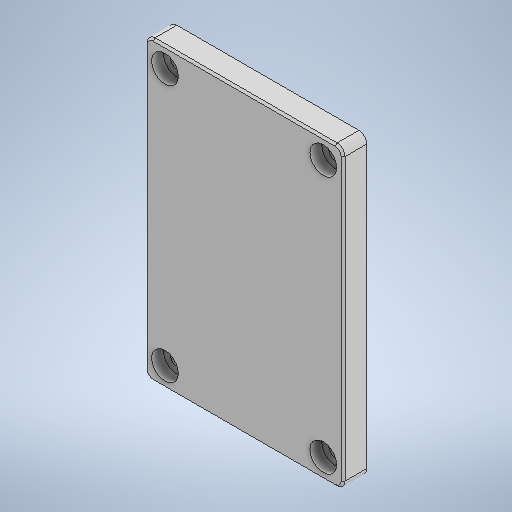
# Autodesk Inventor part: PCB_Cover
Saved by Autodesk Inventor 2025.3 (Build 293356000, 356)
## iProperties
Created: 2025-11-23
Part Number: PCB_Cover
Material: Generic
Document SubType Name: Modeling
Designer: Wula
Density: 1 g/cm^3
Appearance: Default
Author: Wula
Autodesk Inventor part; units mm, degrees
ref_plane "YZ Plane" through (0, 0, 0) normal (1, 0, 0) x (0, 1, 0)
ref_plane "XZ Plane" through (0, 0, 0) normal (0, 1, 0) x (-1, 0, 0)
ref_plane "XY Plane" through (0, 0, 0) normal (0, 0, 1) x (1, 0, 0)
sketch "Sketch1" plane through (0, 0, 0) normal (0, 1, 0) x (-1, 0, 0)
  line L0 (-50, 75) -> (50, 75)
  line L1 (50, 75) -> (50, -75)
  line L2 (50, -75) -> (-50, -75)
  line L3 (-50, -75) -> (-50, 75)
  line L4 (-50, 75) -> (50, -75) construction
  line L5 (50, 75) -> (-50, -75) construction
  point P0 (0, 0)
  dimension "d0" = 150
  dimension "d1" = 100
  constraints: 12 end point, 2 midpoint, 2 parallel, 1 horizontal, 1 perpendicular
  measures "d0" distance of L0.end L1.end
  measures "d1" distance of L1.end L2.end
extrude "Extrusion1" add sketch "Sketch1" along normal blind 12
sketch "Sketch3" plane through (0, 0, 0) normal (0, -1, 0) x (1, 0, 0)
  circle A0 centre (40, 65) radius 7
  circle A1 centre (40, 65) radius 3.25
  line L0 (50, 75) -> (50, -75) projected
  line L1 (-50, 75) -> (50, 75) projected
  circle A2 centre (40, -65) radius 3.25
  circle A3 centre (40, -65) radius 7
  circle A4 centre (-40, 65) radius 3.25
  circle A5 centre (-40, 65) radius 7
  circle A6 centre (-40, -65) radius 3.25
  circle A7 centre (-40, -65) radius 7
  point P0 (0, 0)
  dimension "d4" = 14
  dimension "d5" = 6.5
  dimension "d6" = 10
  dimension "d7" = 10
  dimension "d10" = 130
  dimension "d13" = 80
  constraints: 8 centre point, 4 coincident, 1 horizontal, 1 vertical, 12 other
  measures "d4" diameter of A0
  measures "d5" diameter of A1
  measures "d6" distance from line of L0 A0.centre
  measures "d7" distance from line of L1 A0.centre
  measures "d10" distance of A0.centre A3.centre
  measures "d13" distance of A0.centre A5.centre
hole "Hole1" at (40, 0, 65) at (40, 0, -65) at (-40, 0, 65) at (-40, 0, -65) direction (0, 1, 0) diameter 6.5 end through all counterbore diameter 13.5 counterbore depth 6
fillet "Fillet1" radius 4 4 edges at (50, 6, 75) (50, 6, -75) (-50, 6, -75) (-50, 6, 75)
chamfer "Chamfer3" distance 1 angle 45 8 edges at (0, 0, 75) (48.8284, 0, 73.8284) (50, 0, 0) (48.8284, 0, -73.8284) (0, 0, -75) (-48.8284, 0, -73.8284) (-50, 0, 0) (-48.8284, 0, 73.8284)
body "Solid1"
